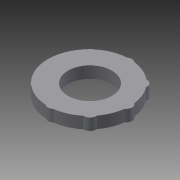
# Autodesk Inventor part: BigGearCenterer
Saved by Autodesk Inventor 2015 (Build 190159000, 159)
## iProperties
Created: 2017-03-08
Part Number: BigGearCenterer
Material: Generic
Document SubType Name: Modeling
Designer: Ernest
Density: 1 g/cm^3
Appearance: Default
Author: Ernest
Autodesk Inventor part; units mm, degrees
ref_plane "YZ Plane" through (0, 0, 0) normal (1, 0, 0) x (0, 1, 0)
ref_plane "XZ Plane" through (0, 0, 0) normal (0, 1, 0) x (-1, 0, 0)
ref_plane "XY Plane" through (0, 0, 0) normal (0, 0, 1) x (1, 0, 0)
sketch "Sketch1" plane through (0, 0, 0) normal (0, 0, 1) x (1, 0, 0)
  circle A0 centre (0, 0) radius 8.75
  circle A1 centre (0.25, 0) radius 24.8
  circle A2 centre (0.25, 0) radius 4.7
  circle A3 centre (-7.45, 0) radius 1.3
  circle A4 centre (-5.1947, -5.4447) radius 1.3
  circle A5 centre (0.25, -7.7) radius 1.3
  circle A6 centre (5.6947, -5.4447) radius 1.3
  circle A7 centre (7.95, 0) radius 1.3
  circle A8 centre (5.6947, 5.4447) radius 1.3
  circle A9 centre (0.25, 7.7) radius 1.3
  circle A10 centre (-5.1947, 5.4447) radius 1.3
  dimension "d0" = 17.5
  dimension "d1" = 49.6
  dimension "d3" = 9.4
  dimension "d4" = 2.6
  dimension "d7" = 360
  constraints: 11 centre point, 2 coincident, 1 tangent, 17 other
  measures "d0" diameter of A0
  measures "d1" diameter of A1
  measures "d3" diameter of A2
  measures "d4" diameter of A3
extrude "Extrusion1" add sketch "Sketch1" along normal blind 2.5 contours A0 A7 | A0 A7 | A3 | A7 A0 A6 A5 A4 A10 A9 A8 | A8 A0 | A0 A8 | A6 A0 | A0 A6 | A9 A0 | A0 A9 | A5 A0 | A0 A5 | A10 A0 | A0 A10 | A4 A0 | A0 A4
body "Solid1"
